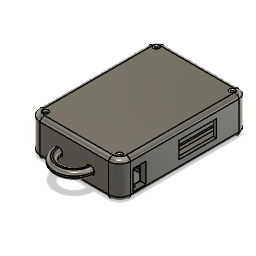
F3KStopWatch (Autodesk Fusion 360 design; units mm, degrees)
Autodesk Fusion 360 part; units mm, degrees
sketch "Sketch1" plane through (0, 0, 0) normal (0, 1, 0) x (1, 0, 0)
  line L0 (-7, 0) -> (-50, 0)
  line L1 (-57, 7) -> (-57, 75)
  line L2 (-52, 80) -> (-5, 80)
  line L3 (0, 75) -> (0, 7)
  line L4 (-57, 80) -> (0, 0) construction
  line L5 (0, 80) -> (-57, 0) construction
  line L6 (-50, 78) -> (-7, 78)
  line L7 (-2, 73) -> (-2, 9)
  line L8 (-9, 2) -> (-48, 2)
  line L9 (-55, 9) -> (-55, 73)
  line L10 (-55, 78) -> (-2, 2) construction
  line L11 (-2, 78) -> (-55, 2) construction
  line L12 (-28.5, 40) -> (-28.5, 88.1661) construction
  line L13 (-43.5, 66.1119) -> (-13.5, 66.1119)
  line L14 (-13.5, 66.1119) -> (-13.5, 26.1119)
  line L15 (-13.5, 26.1119) -> (-43.5, 26.1119)
  line L16 (-43.5, 26.1119) -> (-43.5, 66.1119)
  line L17 (-43.5, 66.1119) -> (-13.5, 26.1119) construction
  line L18 (-13.5, 66.1119) -> (-43.5, 26.1119) construction
  arc A0 (-55, 9) -> (-48, 2) centre (-48, 9) ccw
  arc A1 (-9, 2) -> (-2, 9) centre (-9, 9) ccw
  arc A2 (-2, 73) -> (-7, 78) centre (-7, 73) ccw
  arc A3 (-50, 78) -> (-55, 73) centre (-50, 73) ccw
  arc A4 (-57, 7) -> (-50, 0) centre (-50, 7) ccw
  arc A5 (-7, 0) -> (0, 7) centre (-7, 7) ccw
  arc A6 (0, 75) -> (-5, 80) centre (-5, 75) ccw
  arc A7 (-52, 80) -> (-57, 75) centre (-52, 75) ccw
  point P0 (-28.5, 40)
  point P1 (-28.5, 46.1119)
  dimension "d1" = 57
  dimension "d2" = 80
  dimension "d3" = 53
  dimension "d4" = 76
  dimension "d5" = 30
  dimension "d6" = 40
  dimension "d11" = 7
  dimension "d12" = 7
  dimension "d13" = 5
  dimension "d14" = 5
  dimension "d15" = 7
  dimension "d16" = 7
  dimension "d17" = 5
  dimension "d18" = 5
  constraint horizontal L0
  constraint vertical L1
  constraint horizontal L2
  constraint vertical L3
  constraint coincident L4.end origin
  constraint horizontal L6
  constraint perpendicular L6 L7
  constraint parallel L6 L8
  constraint parallel L7 L9
  constraint coincident L10 P0
  constraint coincident L11 P0
  constraint midpoint L4 P0
  constraint coincident P0 L12.start
  constraint perpendicular L2 L12
  constraint horizontal L13
  constraint perpendicular L13 L14
  constraint parallel L13 L15
  constraint parallel L14 L16
  constraint coincident L17 P1
  constraint coincident L18 P1
  constraint coincident L12 P1
  constraint coincident L11.end L8
  constraint coincident L11.end L9
  constraint tangent L8 A0
  constraint tangent L9 A0
  constraint coincident L10.end L8
  constraint coincident L10.end L7
  constraint tangent L8 A1
  constraint tangent L7 A1
  constraint coincident L11.start L7
  constraint coincident L11.start L6
  constraint tangent L7 A2
  constraint tangent L6 A2
  constraint coincident L10.start L9
  constraint coincident L10.start L6
  constraint tangent L9 A3
  constraint tangent L6 A3
  constraint coincident L5.end L0
  constraint coincident L5.end L1
  constraint tangent L0 A4
  constraint tangent L1 A4
  constraint coincident L4.end L0
  constraint coincident L4.end L3
  constraint tangent L0 A5
  constraint tangent L3 A5
  constraint coincident L5.start L3
  constraint coincident L5.start L2
  constraint tangent L3 A6
  constraint tangent L2 A6
  constraint coincident L4.start L1
  constraint coincident L4.start L2
  constraint tangent L1 A7
  constraint tangent L2 A7
  measures "d1" distance of L4.end L5.end
  measures "d2" distance of L4.end L5.start
  measures "d3" distance of L10.end L11.end
  measures "d4" distance of L11.start L10.end
  measures "d5" distance of L14.end L15.end
  measures "d6" distance of L13.end L14.end
  measures "d11" radius of A0
  measures "d12" radius of A1
  measures "d13" radius of A2
  measures "d14" radius of A3 P0
  measures "d15" radius of A4
  measures "d16" radius of A5
  measures "d17" radius of A6
  measures "d18" radius of A7
  measures "d154" distance of P0
  measures "d155" distance of P0
extrude "Extrude1" add sketch "Sketch1" along normal blind 2 contours L6 L7 L8 L9 A0 A1 A2 A3 makes body 1
extrude "Extrude2" add sketch "Sketch1" along normal blind 21 contours L0 L1 L2 L3 A4 A5 A6 A7 bodies 1
sketch "Sketch3" plane through (0, 0, 0) normal (0, 0, 1) x (1, 0, 0)
  circle A0 centre (40.5808, 13.4916) radius 7.15
  dimension "d19" = 14.3
  measures "d19" diameter of A0
extrude "Extrude3" add sketch "Sketch3" along normal blind 50 separate body makes body 2
move_body "Move1" bodies 2 to x (1, 0, 0) y (0, 1, 0) z (0, 0, 1) at (-26.5696, 0, -50.0846)
move_body "Move2" bodies 2 to x (0, 0, -1) y (0, 1, 0) z (1, 0, 0) at (0, 0, 0)
move_body "Move3" bodies 2 to x (1, 0, 0) y (0, 1, 0) z (0, 0, 1) at (-3.3834, 0, 1.3731)
move_body "Move4" bodies 2 to x (1, 0, 0) y (0, 1, 0) z (0, 0, 1) at (0, -5, 0)
chamfer "Chamfer1" distance 1.5 angle 45 4 edges at (-28.5, 0, -66.1119) (-13.5, 0, -46.1119) (-28.5, 0, -26.1119) (-43.5, 0, -46.1119) on bodies 1
sketch "Sketch4" plane through (0, 0, 0) normal (0, -1, 0) x (1, 0, 0)
  arc A0 (-5, -80) -> (0, -75) centre (-5, -75) ccw
  line L0 (0, -75) -> (0, -7)
  arc A1 (0, -7) -> (-7, 0) centre (-7, -7) ccw
  line L1 (-7, 0) -> (-50, 0)
  arc A2 (-50, 0) -> (-57, -7) centre (-50, -7) ccw
  line L2 (-57, -7) -> (-57, -75)
  arc A3 (-57, -75) -> (-52, -80) centre (-52, -75) ccw
  line L3 (-52, -80) -> (-5, -80)
  line L4 (-45, -24.6119) -> (-12, -24.6119)
  line L5 (-12, -24.6119) -> (-12, -67.6119)
  line L6 (-12, -67.6119) -> (-45, -67.6119)
  line L7 (-45, -67.6119) -> (-45, -24.6119)
  line L8 (-56.9925, -74.7266) -> (-56.9747, 28.4183) construction
  line L9 (0, -61.3272) -> (0, 32.8277) construction
  line L10 (-40.3582, 0) -> (-91.9722, 0) construction
  line L11 (-40.3582, 0) -> (18.5742, 0) construction
  circle A4 centre (-28.5, 0) radius 12.5
  circle A5 centre (-28.5, 0) radius 7.5
  dimension "d24" = 25
  dimension "d25" = 15
  constraint coincident A3 L8.start
  constraint coincident L0 L9.start
  constraint parallel L0 L9
  constraint coincident L1 L10.start
  constraint parallel L1 L10
  constraint perpendicular L9 L11
  constraint midpoint L1 A4.centre
  constraint concentric A4 A5
  measures "d24" diameter of A4
  measures "d25" diameter of A5
extrude "Extrude4" add sketch "Sketch4" along normal blind -13 and the other way blind 8 contours L1 A4 A5 picked at (-39.2868, 0.621) bodies 1
fillet "Fillet1" radius 3 8 edges at (-2.0503, 0, -2.0503) (-28.5, 0, 0) (-54.9497, 0, -2.0503) (-57, 0, -41) (-55.5355, 0, -78.5355) (-28.5, 0, -80) (-1.4645, 0, -78.5355) (0, 0, -41) on bodies 1
fillet "Fillet2" radius 2 8 edges at (-28.5, 2, -78) (-53.5355, 2, -76.5355) (-55, 2, -41) (-52.9497, 2, -4.0503) (-28.5, 2, -2) (-4.0503, 2, -4.0503) (-2, 2, -41) (-3.4645, 2, -76.5355) on bodies 1
fillet "Fillet3" radius 2 4 edges at (-28.5, 8, 7.5) (-28.5, 8, 12.5) (-28.5, 13, 12.5) (-28.5, 13, 7.5) on bodies 1
sketch "Sketch5" plane through (0, 2, 0) normal (0, 1, 0) x (-1, 0, 0)
  line L0 (13.5, -26.1119) -> (43.5, -26.1119)
  line L1 (43.5, -26.1119) -> (43.5, -66.1119)
  line L2 (43.5, -66.1119) -> (13.5, -66.1119)
  line L3 (13.5, -66.1119) -> (13.5, -26.1119)
  line L4 (7, -76) -> (50, -76)
  arc A0 (50, -76) -> (53, -73) centre (50, -73) ccw
  line L5 (53, -73) -> (53, -9)
  arc A1 (53, -9) -> (48, -4) centre (48, -9) ccw
  line L6 (48, -4) -> (9, -4)
  arc A2 (9, -4) -> (4, -9) centre (9, -9) ccw
  line L7 (4, -9) -> (4, -73)
  arc A3 (4, -73) -> (7, -76) centre (7, -73) ccw
  line L8 (30.7713, -66.1119) -> (30.7713, -72.1119) construction
  line L9 (30.7713, -72.1119) -> (8.1959, -72.1119) construction
  line L10 (30.7713, -72.1119) -> (48, -72.1119) construction
  line L11 (43.5, -66.1119) -> (13.5, -26.1119) construction
  line L12 (13.5, -66.1119) -> (43.5, -26.1119) construction
  line L13 (28.5, -46.1119) -> (28.5, -82.7319)
  line L14 (28.5, -46.1119) -> (28.5, -15.5457) construction
  line L15 (28.5, -72.1119) -> (10.8, -72.1119)
  line L16 (28.5, -72.1119) -> (46.2, -72.1119)
  line L17 (28.5, -26.1119) -> (28.5, -23.4119) construction
  line L18 (28.5, -23.4119) -> (46.2, -23.4119)
  line L19 (28.5, -23.4119) -> (10.8, -23.4119)
  line L20 (46.2, -72.1119) -> (46.2, -23.4119)
  line L21 (10.8, -72.1119) -> (10.8, -23.4119)
  line L22 (28.5, -22.4119) -> (9.8, -22.4119)
  line L23 (9.8, -73.1119) -> (9.8, -22.4119)
  line L24 (28.5, -73.1119) -> (9.8, -73.1119)
  line L25 (28.5, -73.1119) -> (47.2, -73.1119)
  line L26 (47.2, -73.1119) -> (47.2, -22.4119)
  line L27 (28.5, -22.4119) -> (47.2, -22.4119)
  line L28 (46.2, -72.1119) -> (42.2, -72.1119)
  line L29 (42.2, -72.1119) -> (42.2, -73.1119)
  line L30 (10.8, -72.1119) -> (15.8, -72.1119)
  line L31 (15.8, -72.1119) -> (15.8, -73.1119)
  line L32 (46.2, -23.4119) -> (41.2, -23.4119)
  line L33 (41.2, -23.4119) -> (41.2, -22.4119)
  line L34 (10.8, -23.4119) -> (15.8, -23.4119)
  line L35 (15.8, -23.4119) -> (15.8, -22.4119)
  dimension "d36" = 6
  dimension "d37" = 17.7
  dimension "d38" = 17.7
  dimension "d39" = 2.7
  dimension "d40" = 17.7
  dimension "d41" = 17.7
  dimension "d42" = 1
  dimension "d45" = 4
  dimension "d46" = 5
  dimension "d47" = 5
  dimension "d48" = 5
  constraint coincident L2 L8.start
  constraint perpendicular L2 L8
  constraint perpendicular L8 L9
  constraint perpendicular L8 L10
  constraint coincident L1.end L2.start
  constraint coincident L0.start L3.end
  constraint coincident L2.end L3.start
  constraint coincident L0.end L1.start
  constraint midpoint L11 L13.start
  constraint perpendicular L4 L13
  constraint perpendicular L0 L14
  constraint coincident L13 L15.start
  constraint coincident L9 L15.start
  constraint perpendicular L13 L15
  constraint perpendicular L8 L16
  constraint midpoint L0 L17.start
  constraint perpendicular L0 L17
  constraint perpendicular L1 L18
  constraint perpendicular L14 L19
  constraint perpendicular L20 L28
  constraint coincident L25 L29.end
  constraint perpendicular L25 L29
  constraint perpendicular L21 L30
  constraint coincident L24 L31.end
  constraint perpendicular L24 L31
  constraint perpendicular L20 L32
  constraint coincident L27 L33.end
  constraint perpendicular L27 L33
  constraint perpendicular L21 L34
  constraint coincident L22 L35.end
  constraint perpendicular L22 L35
  measures "d36" distance of L8.start L8.end
  measures "d37" distance of L15.start L15.end
  measures "d38" distance of L15.start L16.end
  measures "d39" distance of L17.start L17.end
  measures "d40" distance of L17.end L18.end
  measures "d41" distance of L17.end L19.end
  measures "d45" distance of L16.end L28.end
  measures "d46" distance of L15.end L30.end
  measures "d47" distance of L18.end L32.end
  measures "d48" distance of L19.end L34.end
extrude "Extrude5" add sketch "Sketch5" along normal blind 2 contours L13 L16 L25 L29 | L13 L15 L24 L31 | L15 L19 L21 L22 L23 L24 L30 L31 L34 L35 | L16 L18 L20 L25 L26 L27 L28 L29 L32 L33 | L18 L19 L22 L27 L33 L35 bodies 1
extrude "Extrude6" cut sketch "Sketch5" along normal blind 2 contours L13 L16 L25 L29 | L13 L15 L24 L31 | L18 L19 L22 L27 L33 L35 bodies 1
move_body "Move5" bodies 2 to x (1, 0, 0) y (0, 1, 0) z (0, 0, 1) at (0, 0.8294, 0.1037)
move_body "Move6" bodies 2 to x (1, 0, 0) y (0, 1, 0) z (0, 0, 1) at (0, 0, 0.5)
sketch "Sketch8" plane through (0, 0, 0) normal (0, 1, 0) x (1, 0, 0)
  line L0 (28.9998, 41.3515) -> (63.9998, 41.3515)
  line L1 (63.9998, 41.3515) -> (63.9998, -6.6485)
  line L2 (63.9998, -6.6485) -> (28.9998, -6.6485)
  line L3 (28.9998, -6.6485) -> (28.9998, 41.3515)
  line L4 (28.9998, 41.3515) -> (63.9998, -6.6485) construction
  line L5 (63.9998, 41.3515) -> (28.9998, -6.6485) construction
  line L6 (63.9998, -10.1485) -> (28.9998, -10.1485)
  line L7 (28.9998, -10.1485) -> (28.9998, 44.8515)
  line L8 (28.9998, 44.8515) -> (63.9998, 44.8515)
  line L9 (63.9998, 44.8515) -> (63.9998, -10.1485)
  line L10 (63.9998, -10.1485) -> (28.9998, 44.8515) construction
  line L11 (28.9998, -10.1485) -> (63.9998, 44.8515) construction
  line L12 (56.9998, -8.6485) -> (35.9998, -8.6485)
  line L13 (35.9998, -8.6485) -> (35.9998, 43.3515)
  line L14 (35.9998, 43.3515) -> (56.9998, 43.3515)
  line L15 (56.9998, 43.3515) -> (56.9998, -8.6485)
  line L16 (56.9998, -8.6485) -> (35.9998, 43.3515) construction
  line L17 (35.9998, -8.6485) -> (56.9998, 43.3515) construction
  point P0 (46.4998, 17.3515)
  point P1 (46.4998, 17.3515)
  dimension "d63" = 35
  dimension "d64" = 48
  dimension "d65" = 35
  dimension "d66" = 55
  dimension "d67" = 21
  dimension "d68" = 52
  constraint horizontal L0
  constraint vertical L1
  constraint horizontal L2
  constraint vertical L3
  constraint horizontal L6
  constraint perpendicular L6 L7
  constraint parallel L6 L8
  constraint parallel L7 L9
  constraint coincident L10 P1
  constraint coincident L11 P1
  constraint midpoint L5 P1
  constraint horizontal L12
  constraint perpendicular L12 L13
  constraint parallel L12 L14
  constraint parallel L13 L15
  constraint coincident L16 P1
  constraint coincident L17 P1
  constraint coincident P1 P0
  measures "d63" distance of L0.start L0.end
  measures "d64" distance of L0.start L2.end
  measures "d65" distance of L7.end L8.end
  measures "d66" distance of L6.end L7.end
  measures "d67" distance of L13.end L14.end
  measures "d68" distance of L12.end L13.end
extrude "Extrude8" add sketch "Sketch8" along normal blind 16.5 and the other way blind -3.1 separate body contours L0 L13 L14 L15 | L0 L2 L13 L15 | L2 L12 L13 L15 makes body 3
extrude "Extrude9" add sketch "Sketch8" along normal blind 3.1 separate body contours L0 L2 L3 L7 L13 | L0 L2 L13 L15 | L0 L1 L2 L9 L15 makes body 4
extrude "Extrude10" add sketch "Sketch8" along normal blind 4.9 and the other way blind -3.1 separate body makes body 5
combine "Combine1" operation add target body 3 tool bodies 4 5 keep tools
combine "Combine2" operation add target body 4 tool bodies 3 5 keep tools
combine "Combine3" operation add target body 3 tool bodies 4 5 keep tools
combine "Combine4" operation add target body 3 tool bodies 5 keep tools
combine "Combine5" operation add target body 3 tool bodies 4 keep tools
delete_body "RemoveBody1" bodies 4
delete_body "RemoveBody2" bodies 5
move_body "Move7" bodies 3 to x (1, 0, 0) y (0, 1, 0) z (0, 0, 1) at (-75.2922, 0, -30.8262)
move_body "Move8" bodies 3 to x (1, 0, 0) y (0, 1, 0) z (0, 0, 1) at (0, 2, 0)
move_body "Move9" bodies 3 to x (1, 0, 0) y (0, 1, 0) z (0, 0, 1) at (0, 0, 0.4)
move_body "Move10" bodies 3 to x (1, 0, 0) y (0, 1, 0) z (0, 0, 1) at (0.3, 0, 0)
move_body "Move11" bodies 2 to x (0, 0, 1) y (0, 1, 0) z (-1, 0, 0) at (0, 0, 0)
move_body "Move12" bodies 2 to x (1, 0, 0) y (0, 1, 0) z (0, 0, 1) at (-58.8123, 0, -12.8386)
move_body "Move13" bodies 2 to x (1, 0, 0) y (0, 1, 0) z (0, 0, 1) at (-1.1, 4.5, 0)
sketch "Sketch9" plane through (0, 0, 0) normal (1, 0, 0) x (0, 0, -1)
  line L0 (7, 3) -> (75, 3)
  line L1 (75, 3) -> (75, 21)
  line L2 (75, 21) -> (7, 21)
  line L3 (7, 21) -> (7, 3)
  line L4 (75, 12) -> (49, 12) construction
  line L5 (60.75, 6.75) -> (37.25, 6.75)
  line L6 (37.25, 6.75) -> (37.25, 17.25)
  line L7 (37.25, 17.25) -> (60.75, 17.25)
  line L8 (60.75, 17.25) -> (60.75, 6.75)
  line L9 (60.75, 6.75) -> (37.25, 17.25) construction
  line L10 (37.25, 6.75) -> (60.75, 17.25) construction
  point P0 (49, 12)
  dimension "d80" = 26
  dimension "d81" = 23.5
  dimension "d82" = 10.5
  constraint midpoint L1 L4.start
  constraint perpendicular L1 L4
  constraint horizontal L5
  constraint perpendicular L5 L6
  constraint parallel L5 L7
  constraint parallel L6 L8
  constraint coincident L9 P0
  constraint coincident L10 P0
  constraint coincident P0 L4.end
  measures "d80" distance of L4.start P0
  measures "d81" distance of L6.end L7.end
  measures "d82" distance of L5.end L6.end
extrude "Extrude11" cut sketch "Sketch9" against normal blind 3 contours L5 L6 L7 L8 bodies 1
sketch "Sketch10" plane through (0, 2, 0) normal (0, 1, 0) x (-1, 0, 0)
  line L0 (41.2, -22.4119) -> (47.2, -22.4119)
  line L1 (47.2, -22.4119) -> (47.2, -73.1119)
  line L2 (47.2, -73.1119) -> (42.2, -73.1119)
  line L3 (42.2, -73.1119) -> (42.2, -72.1119)
  line L4 (42.2, -72.1119) -> (46.2, -72.1119)
  line L5 (46.2, -72.1119) -> (46.2, -23.4119)
  line L6 (46.2, -23.4119) -> (41.2, -23.4119)
  line L7 (41.2, -23.4119) -> (41.2, -22.4119)
  line L8 (13.5, -26.1119) -> (43.5, -26.1119)
  line L9 (43.5, -26.1119) -> (43.5, -66.1119)
  line L10 (43.5, -66.1119) -> (13.5, -66.1119)
  line L11 (13.5, -66.1119) -> (13.5, -26.1119)
  line L12 (7, -76) -> (50, -76)
  arc A0 (50, -76) -> (53, -73) centre (50, -73) ccw
  line L13 (53, -73) -> (53, -9)
  arc A1 (53, -9) -> (48, -4) centre (48, -9) ccw
  line L14 (48, -4) -> (9, -4)
  arc A2 (9, -4) -> (4, -9) centre (9, -9) ccw
  line L15 (4, -9) -> (4, -73)
  arc A3 (4, -73) -> (7, -76) centre (7, -73) ccw
  line L16 (15.8, -22.4119) -> (15.8, -23.4119)
  line L17 (15.8, -23.4119) -> (10.8, -23.4119)
  line L18 (10.8, -23.4119) -> (10.8, -72.1119)
  line L19 (10.8, -72.1119) -> (15.8, -72.1119)
  line L20 (15.8, -72.1119) -> (15.8, -73.1119)
  line L21 (15.8, -73.1119) -> (9.8, -73.1119)
  line L22 (9.8, -73.1119) -> (9.8, -22.4119)
  line L23 (9.8, -22.4119) -> (15.8, -22.4119)
  line L24 (42.4256, -4) -> (42.4256, -16.2447) construction
  line L25 (50.4256, -6.1223) -> (34.4256, -6.1223)
  line L26 (34.4256, -6.1223) -> (34.4256, -14.1223)
  line L27 (34.4256, -14.1223) -> (50.4256, -14.1223)
  line L28 (50.4256, -14.1223) -> (50.4256, -6.1223)
  line L29 (50.4256, -6.1223) -> (34.4256, -14.1223) construction
  line L30 (34.4256, -6.1223) -> (50.4256, -14.1223) construction
  point P0 (42.4256, -10.1223)
  dimension "d85" = 16
  dimension "d86" = 8
  constraint coincident L14 L24.start
  constraint perpendicular L14 L24
  constraint horizontal L25
  constraint perpendicular L25 L26
  constraint parallel L25 L27
  constraint parallel L26 L28
  constraint coincident L29 P0
  constraint coincident L30 P0
  constraint midpoint L24 P0
  measures "d85" distance of L26.end L27.end
  measures "d86" distance of L25.end L26.end
extrude "Extrude12" cut sketch "Sketch10" against normal blind 9 contours L25 L26 L27 L28 bodies 1
sketch "Sketch15" plane through (0, 2, 0) normal (0, 1, 0) x (-1, 0, 0)
  line L0 (34.4256, -6.1223) -> (50.4256, -6.1223)
  line L1 (50.4256, -6.1223) -> (50.4256, -14.1223)
  line L2 (50.4256, -14.1223) -> (34.4256, -14.1223)
  line L3 (34.4256, -14.1223) -> (34.4256, -6.1223)
  line L4 (41.2, -22.4119) -> (47.2, -22.4119)
  line L5 (47.2, -22.4119) -> (47.2, -73.1119)
  line L6 (47.2, -73.1119) -> (42.2, -73.1119)
  line L7 (42.2, -73.1119) -> (42.2, -72.1119)
  line L8 (42.2, -72.1119) -> (46.2, -72.1119)
  line L9 (46.2, -72.1119) -> (46.2, -23.4119)
  line L10 (46.2, -23.4119) -> (41.2, -23.4119)
  line L11 (41.2, -23.4119) -> (41.2, -22.4119)
  line L12 (13.5, -26.1119) -> (43.5, -26.1119)
  line L13 (43.5, -26.1119) -> (43.5, -66.1119)
  line L14 (43.5, -66.1119) -> (13.5, -66.1119)
  line L15 (13.5, -66.1119) -> (13.5, -26.1119)
  line L16 (7, -76) -> (50, -76)
  arc A0 (50, -76) -> (53, -73) centre (50, -73) ccw
  line L17 (53, -73) -> (53, -9)
  arc A1 (53, -9) -> (48, -4) centre (48, -9) ccw
  line L18 (48, -4) -> (9, -4)
  arc A2 (9, -4) -> (4, -9) centre (9, -9) ccw
  line L19 (4, -9) -> (4, -73)
  arc A3 (4, -73) -> (7, -76) centre (7, -73) ccw
  line L20 (15.8, -22.4119) -> (15.8, -23.4119)
  line L21 (15.8, -23.4119) -> (10.8, -23.4119)
  line L22 (10.8, -23.4119) -> (10.8, -72.1119)
  line L23 (10.8, -72.1119) -> (15.8, -72.1119)
  line L24 (15.8, -72.1119) -> (15.8, -73.1119)
  line L25 (15.8, -73.1119) -> (9.8, -73.1119)
  line L26 (9.8, -73.1119) -> (9.8, -22.4119)
  line L27 (9.8, -22.4119) -> (15.8, -22.4119)
  line L28 (4, -9) -> (31.5949, -9) construction
  line L29 (4, -9) -> (-8.1404, -9) construction
  line L30 (4, -9) -> (25, -9)
  line L31 (25, -9) -> (25, -1.0306)
  line L32 (4, -9) -> (2.2, -9)
  line L33 (25, -1.0306) -> (-6.9566, -1.0306) construction
  line L34 (2.2, -9) -> (2.2, -7.0306)
  line L35 (2.2, -1.0306) -> (25, -1.0306)
  line L36 (25, -1.0306) -> (8.2, -1.0306)
  arc A4 (8.2, -1.0306) -> (2.2, -7.0306) centre (8.2, -7.0306) ccw
  dimension "d107" = 21
  dimension "d113" = 1.8
  dimension "d114" = 6
  constraint coincident A2.end L19.start
  constraint perpendicular L19 L28
  constraint perpendicular L19 L29
  constraint perpendicular L19 L30
  constraint perpendicular L18 L31
  constraint perpendicular L19 L32
  constraint perpendicular L31 L33
  constraint coincident L33 L35.start
  constraint perpendicular L33 L34
  constraint coincident L35.start L34
  constraint coincident L35.start L36
  constraint tangent L34 A4
  constraint tangent L36 A4
  measures "d107" distance of A2.end L30.end
  measures "d113" distance of A2.end L32.end
  measures "d114" radius of A4
extrude "Extrude18" add sketch "Sketch15" along normal blind 18 separate body contours L18 A2 L31 L32 L34 L35 L36 A4 | L18 A2 L30 L31 makes body 6
move_body "Move14" bodies 6 to x (1, 0, 0) y (0, 1, 0) z (0, 0, 1) at (2, 0, 0)
fillet "Fillet7" [no effect]
combine "Combine7" operation add target body 1 tool bodies 6 keep tools
delete_body "RemoveBody3" bodies 6
fillet "Fillet8" radius 1 5 edges at (-23, 11, -9) (-23, 12, -2) (-23, 2.5858, -2.5858) (-23, 2, -6.5) (-23, 20, -5.5) on bodies 1
fillet "Fillet9" radius 1 2 edges at (-12, 20, -9) (-22.7071, 19.7071, -8.7071) on bodies 1
sketch "Sketch16" plane through (-2, 0, 0) normal (-1, 0, 0) x (0, 0, 1)
  line L0 (-37.25, 17.25) -> (-37.25, 6.75)
  line L1 (-37.25, 6.75) -> (-60.75, 6.75)
  line L2 (-60.75, 6.75) -> (-60.75, 17.25)
  line L3 (-60.75, 17.25) -> (-37.25, 17.25)
  line L4 (-73, 4) -> (-9, 4)
  line L5 (-9, 4) -> (-9, 19)
  line L6 (-9, 19) -> (-9, 21)
  line L7 (-9, 21) -> (-73, 21)
  line L8 (-73, 21) -> (-73, 4)
  line L9 (-9, -0.9635) -> (-9, 21) construction
  line L10 (-9, 10.0182) -> (-22.3565, 10.0182) construction
  line L11 (-9, 10.0182) -> (-10.5, 10.0182) construction
  line L12 (-10.5, 10.0182) -> (-14.5, 10.0182) construction
  line L13 (-14.5, 10.0182) -> (-12.5, 10.0182) construction
  line L14 (-14.75, 14.5182) -> (-10.25, 14.5182)
  line L15 (-10.25, 14.5182) -> (-10.25, 5.5182)
  line L16 (-10.25, 5.5182) -> (-14.75, 5.5182)
  line L17 (-14.75, 5.5182) -> (-14.75, 14.5182)
  line L18 (-14.75, 14.5182) -> (-10.25, 5.5182) construction
  line L19 (-10.25, 14.5182) -> (-14.75, 5.5182) construction
  point P0 (-12.5, 10.0182)
  dimension "d119" = 13.3565
  dimension "d120" = 1.5
  dimension "d121" = 4
  dimension "d122" = 4.5
  dimension "d123" = 9
  constraint coincident L6.end L7.start
  constraint perpendicular L7 L9
  constraint midpoint L9 L10.start
  constraint perpendicular L9 L10
  constraint perpendicular L5 L11
  constraint perpendicular L9 L12
  constraint midpoint L12 P0
  constraint horizontal L14
  constraint perpendicular L14 L15
  constraint parallel L14 L16
  constraint parallel L15 L17
  constraint coincident L18 P0
  constraint coincident L19 P0
  constraint coincident P0 L13.end
  measures "d119" distance of L10.start L10.end
  measures "d120" distance of L10.start L11.end
  measures "d121" distance of L11.end L12.end
  measures "d122" distance of L15.end L16.end
  measures "d123" distance of L14.end L15.end
extrude "Extrude19" cut sketch "Sketch16" against normal blind 4 contours L14 L15 L16 L17 bodies 1
chamfer "Chamfer2" distance 1.8 angle 45 4 edges at (0, 14.5182, -12.5) (0, 10.0182, -14.75) (0, 5.5182, -12.5) (0, 10.0182, -10.25) on bodies 1
sketch "Sketch17" plane through (0, 0, -2) normal (0, 0, -1) x (-1, 0, 0)
  line L0 (24, 19) -> (24, 4)
  line L1 (24, 4) -> (48, 4)
  line L2 (48, 4) -> (48, 21)
  line L3 (48, 21) -> (9, 21)
  line L4 (9, 21) -> (9, 20)
  line L5 (9, 20) -> (22.2679, 20)
  spline S0 degree 3 poles (22.2679, 20) (22.5228, 20) (22.8153, 19.9104) (23.3848, 19.6039) (23.7229, 19.2771) (24, 19) knots 0.505532 0.505532 0.505532 0.505532 0.581995 0.581995 0.699558 0.699558 0.699558 0.699558
  line L6 (55.8373, 1.7757) -> (46.5836, 1.7757)
  line L7 (46.5836, 1.7757) -> (46.5836, 12.5)
  line L8 (46.5836, 12.5) -> (55.8373, 12.5)
  line L9 (55.8373, 12.5) -> (55.8373, 1.7757)
  dimension "d127" = 9.2536
  constraint horizontal L6
  constraint vertical L7
  constraint horizontal L8
  constraint vertical L9
  measures "d127" distance of L6.start L6.end
extrude "Extrude20" add sketch "Sketch17" along normal blind 65.5 and the other way blind -13 separate body contours L1 L2 L7 L8 | L1 L2 L6 L7 L8 L9 makes body 7
combine "Combine8" operation cut target body 7 tool bodies 2 keep tools
combine "Combine9" operation add target body 1 tool bodies 7 keep tools
delete_body "RemoveBody4" bodies 7
sketch "Sketch18" plane through (0, 2, 0) normal (0, 1, 0) x (-1, 0, 0)
  line L0 (1.0146, -8.9828) -> (25.0146, -8.9828)
  line L1 (25.0146, -8.9828) -> (25.0146, -10.7828)
  line L2 (25.0146, -10.7828) -> (1.0146, -10.7828)
  line L3 (1.0146, -10.7828) -> (1.0146, -8.9828)
  dimension "d132" = 24
  dimension "d133" = 1.8
  constraint horizontal L0
  constraint vertical L1
  constraint horizontal L2
  constraint vertical L3
  measures "d132" distance of L0.start L0.end
  measures "d133" distance of L0.start L2.end
extrude "Extrude21" cut sketch "Sketch18" along normal blind 23 and the other way blind 0 bodies 1
sketch "Sketch19" plane through (0, 0, -80) normal (0, 0, -1) x (-1, 0, 0)
  line L0 (5, 3) -> (52, 3)
  line L1 (52, 3) -> (52, 21)
  line L2 (52, 21) -> (5, 21) construction
  line L3 (5, 21) -> (5, 3)
  line L4 (5, 12) -> (52, 12) construction
  line L5 (5, 12) -> (13, 12)
  line L6 (52, 12) -> (44, 12)
  circle A0 centre (13, 12) radius 6.25
  circle A1 centre (13, 12) radius 8.75 construction
  circle A2 centre (44, 12) radius 8.75 construction
  circle A3 centre (44, 12) radius 6.25
  dimension "d138" = 8
  dimension "d139" = 8
  dimension "d140" = 12.5
  dimension "d141" = 17.5
  dimension "d142" = 17.5
  dimension "d143" = 12.5
  constraint midpoint L3 L4.start
  constraint midpoint L1 L4.end
  constraint perpendicular L3 L5
  constraint perpendicular L1 L6
  constraint coincident L5.end A0.centre
  constraint concentric A0 A1
  constraint coincident L6.end A2.centre
  constraint concentric A2 A3
  measures "d138" distance of L4.start L5.end
  measures "d139" distance of L4.end L6.end
  measures "d140" diameter of A0
  measures "d141" diameter of A1
  measures "d142" diameter of A2
  measures "d143" diameter of A3
extrude "Extrude22" cut sketch "Sketch19" against normal blind 3 bodies 1
sketch "Sketch20" plane through (0, 21, 0) normal (0, 1, 0) x (-1, 0, 0)
  arc A0 (0, -75) -> (5, -80) centre (5, -75) ccw
  line L0 (5, -80) -> (52, -80)
  arc A1 (52, -80) -> (57, -75) centre (52, -75) ccw
  line L1 (57, -75) -> (57, -7)
  arc A2 (57, -7) -> (50, 0) centre (50, -7) ccw
  line L2 (50, 0) -> (7, 0)
  arc A3 (7, 0) -> (0, -7) centre (7, -7) ccw
  line L3 (0, -7) -> (0, -75)
  line L4 (2, -10.7828) -> (1.0146, -10.7828)
  line L5 (1.0146, -10.7828) -> (1.0146, -8.9828)
  line L6 (1.0146, -8.9828) -> (2, -8.9828)
  arc A4 (9, -2) -> (2, -8.9828) centre (9, -9) ccw
  line L7 (9, -2) -> (48, -2)
  arc A5 (55, -9) -> (48, -2) centre (48, -9) ccw
  line L8 (55, -9) -> (55, -73)
  arc A6 (50, -78) -> (55, -73) centre (50, -73) ccw
  line L9 (50, -78) -> (7, -78)
  arc A7 (2, -73) -> (7, -78) centre (7, -73) ccw
  line L10 (2, -73) -> (2, -10.7828)
extrude "Extrude23" add sketch "Sketch20" along normal blind 2 and the other way blind 1 separate body contours A0 L0 A1 L1 A2 L2 A3 L3 | L4 L5 L6 A4 L7 A5 L8 A6 L9 A7 L10 makes body 8
combine "Combine10" operation cut target body 8 tool bodies 1 2 keep tools
fillet "Fillet11" radius 3 8 edges at (-57, 23, -41) (-54.9497, 23, -2.0503) (-28.5, 23, 0) (-2.0503, 23, -2.0503) (0, 23, -41) (-1.4645, 23, -78.5355) (-28.5, 23, -80) (-55.5355, 23, -78.5355) on bodies 8
sketch "Sketch21" plane through (0, 21, 0) normal (0, 1, 0) x (-1, 0, 0)
  arc A0 (0, -75) -> (5, -80) centre (5, -75) ccw
  line L0 (5, -80) -> (52, -80)
  arc A1 (52, -80) -> (57, -75) centre (52, -75) ccw
  line L1 (57, -75) -> (57, -7)
  arc A2 (57, -7) -> (50, 0) centre (50, -7) ccw
  line L2 (50, 0) -> (7, 0)
  arc A3 (7, 0) -> (0, -7) centre (7, -7) ccw
  line L3 (0, -7) -> (0, -75)
  line L4 (2, -10.7828) -> (1.0146, -10.7828)
  line L5 (1.0146, -10.7828) -> (1.0146, -8.9828)
  line L6 (1.0146, -8.9828) -> (2, -8.9828)
  arc A4 (9, -2) -> (2, -8.9828) centre (9, -9) ccw
  line L7 (9, -2) -> (48, -2)
  arc A5 (55, -9) -> (48, -2) centre (48, -9) ccw
  line L8 (55, -9) -> (55, -73)
  arc A6 (50, -78) -> (55, -73) centre (50, -73) ccw
  line L9 (50, -78) -> (7, -78)
  arc A7 (2, -73) -> (7, -78) centre (7, -73) ccw
  line L10 (2, -73) -> (2, -10.7828)
  line L11 (0.9141, -73) -> (4, -73)
  line L12 (7, -76) -> (7, -78.5355)
  line L13 (7, -78.5355) -> (5.9141, -78.5355)
  line L14 (0.9141, -73.5355) -> (0.9141, -73)
  line L15 (50, -78.5355) -> (51, -78.5355)
  line L16 (56, -73.5355) -> (56, -72.5355)
  line L17 (56, -72.5355) -> (53, -72.5355)
  line L18 (50, -75.5355) -> (50, -78.5355)
  line L19 (55.8559, -7.968) -> (54.2906, -7.968)
  line L20 (48.7906, -2.468) -> (48.7906, -0.9027)
  line L21 (48.7906, -0.9027) -> (48.3559, -0.9027)
  line L22 (55.8559, -8.4027) -> (55.8559, -7.968)
  arc A8 (0.9141, -73.5355) -> (5.9141, -78.5355) centre (5.9141, -73.5355) ccw
  arc A9 (51, -78.5355) -> (56, -73.5355) centre (51, -73.5355) ccw
  arc A10 (55.8559, -8.4027) -> (48.3559, -0.9027) centre (48.3559, -8.4027) ccw
  arc A11 (48.7906, -2.468) -> (54.2906, -7.968) centre (54.2906, -2.468) ccw
  arc A12 (53, -72.5355) -> (50, -75.5355) centre (53, -75.5355) ccw
  arc A13 (7, -76) -> (4, -73) centre (4, -76) ccw
  point P0 (56, -78.5355)
  point P1 (50, -72.5355)
  point P2 (48.7906, -7.968)
  dimension "d154" = 6
  dimension "d155" = 6
  dimension "d156" = 7.0653
  dimension "d157" = 5
  dimension "d158" = 5
  dimension "d159" = 7.5
  dimension "d160" = 5.5
  dimension "d161" = 3
  dimension "d162" = 3
  constraint horizontal L11
  constraint vertical L12
  constraint horizontal L13
  constraint vertical L14
  constraint horizontal L15
  constraint vertical L16
  constraint horizontal L17
  constraint vertical L18
  constraint horizontal L19
  constraint vertical L20
  constraint horizontal L21
  constraint vertical L22
  constraint tangent L13 A8
  constraint tangent L14 A8
  constraint coincident P0 L15
  constraint coincident P0 L16
  constraint tangent L15 A9
  constraint tangent L16 A9
  constraint tangent L21 A10
  constraint tangent L22 A10
  constraint coincident P2 L20
  constraint coincident P2 L19
  constraint tangent L20 A11
  constraint tangent L19 A11
  constraint coincident P1 L17
  constraint coincident P1 L18
  constraint tangent L17 A12
  constraint tangent L18 A12
  constraint tangent L11 A13
  constraint tangent L12 A13
  measures "d154" distance of L15.start P0
  measures "d155" distance of L15.start P1
  measures "d156" distance of L19.start P2
  measures "d157" radius of A8
  measures "d158" radius of A9
  measures "d159" radius of A10
  measures "d160" radius of A11
  measures "d161" radius of A12
  measures "d162" radius of A13
extrude "Extrude24" add sketch "Sketch21" along normal blind -7 and the other way blind 1 contours A7 L11 L12 A13 bodies 1
extrude "Extrude25" add sketch "Sketch21" along normal blind -6 and the other way blind 1 contours L8 A6 L17 L18 A12 bodies 1
extrude "Extrude26" add sketch "Sketch21" along normal blind -7 and the other way blind 1 contours A5 L19 L20 A11 bodies 1
fillet "Fillet12" radius 2 9 edges at (-54.6071, 14, -7.968) (-50.4015, 14, -6.3571) (-48.7906, 14, -2.2564) (-3, 14, -73) (-6.1213, 14, -73.8787) (-7, 14, -77) (-50, 15, -76.7678) (-50.8787, 15, -73.4142) (-54, 15, -72.5355) on bodies 1
fillet "Fillet13" radius 1 4 edges at (-50.7918, 12.5, -15) (-46.5836, 7.25, -15) (-50.7918, 12.5, -67.5) (-46.5836, 8.25, -67.5) on bodies 1
sketch "Sketch22" plane through (0, 2, 0) normal (0, 1, 0) x (-1, 0, 0)
  line L0 (4, -10.7828) -> (4, -73)
  arc A0 (4, -73) -> (7, -76) centre (7, -73) ccw
  line L1 (7, -76) -> (50, -76)
  arc A1 (50, -76) -> (53, -73) centre (50, -73) ccw
  line L2 (53, -73) -> (53, -67.5)
  line L3 (53, -67.5) -> (47.5836, -67.5)
  arc A2 (47.2, -67.4235) -> (47.5836, -67.5) centre (47.5836, -66.5) ccw
  line L4 (47.2, -67.4235) -> (47.2, -73.1119)
  line L5 (47.2, -73.1119) -> (42.2, -73.1119)
  line L6 (42.2, -73.1119) -> (42.2, -72.1119)
  line L7 (42.2, -72.1119) -> (46.2, -72.1119)
  line L8 (46.2, -72.1119) -> (46.2, -23.4119)
  line L9 (46.2, -23.4119) -> (41.2, -23.4119)
  line L10 (41.2, -23.4119) -> (41.2, -22.4119)
  line L11 (41.2, -22.4119) -> (46.5836, -22.4119)
  line L12 (46.5836, -22.4119) -> (46.5836, -16)
  arc A3 (47.5836, -15) -> (46.5836, -16) centre (47.5836, -16) ccw
  line L13 (47.5836, -15) -> (53, -15)
  line L14 (53, -15) -> (53, -9)
  arc A4 (53, -9) -> (48, -4) centre (48, -9) ccw
  line L15 (48, -4) -> (24, -4)
  line L16 (24, -4) -> (24, -8)
  spline S0 degree 3 poles (24, -8) (23.7229, -8.2771) (23.3848, -8.6039) (22.8771, -8.8772) (22.6793, -8.9523) (22.4851, -8.9828) knots 0 0 0 0 0.117563 0.117563 0.172976 0.172976 0.172976 0.172976
  line L17 (22.4851, -8.9828) -> (1.0146, -8.9828)
  line L18 (1.0146, -8.9828) -> (1.0146, -10.7828)
  line L19 (1.0146, -10.7828) -> (4, -10.7828)
  line L20 (15.8, -22.4119) -> (15.8, -23.4119)
  line L21 (15.8, -23.4119) -> (10.8, -23.4119)
  line L22 (10.8, -23.4119) -> (10.8, -72.1119)
  line L23 (10.8, -72.1119) -> (15.8, -72.1119)
  line L24 (15.8, -72.1119) -> (15.8, -73.1119)
  line L25 (15.8, -73.1119) -> (9.8, -73.1119)
  line L26 (9.8, -73.1119) -> (9.8, -22.4119)
  line L27 (9.8, -22.4119) -> (15.8, -22.4119)
  line L28 (13.5, -26.1119) -> (43.5, -26.1119)
  line L29 (43.5, -26.1119) -> (43.5, -66.1119)
  line L30 (43.5, -66.1119) -> (13.5, -66.1119)
  line L31 (13.5, -66.1119) -> (13.5, -26.1119)
  line L32 (34.4256, -6.1223) -> (50.4256, -6.1223)
  line L33 (50.4256, -6.1223) -> (50.4256, -14.1223)
  line L34 (50.4256, -14.1223) -> (34.4256, -14.1223)
  line L35 (34.4256, -14.1223) -> (34.4256, -6.1223)
  line L36 (4, -10.7828) -> (23.8799, -10.7828) construction
  line L37 (1.0146, -10.7828) -> (14.0146, -10.7828) construction
  line L38 (14.0146, -10.7828) -> (19.0146, -10.7828)
  line L39 (19.0146, -10.7828) -> (19.0146, -11.7828)
  line L40 (19.0146, -11.7828) -> (14.0146, -11.7828)
  line L41 (14.0146, -11.7828) -> (14.0146, -10.7828)
  dimension "d179" = 13
  dimension "d180" = 5
  dimension "d181" = 1
  constraint coincident L0.start L19.end
  constraint perpendicular L0 L36
  constraint coincident L18.end L19.start
  constraint perpendicular L18 L37
  constraint horizontal L38
  constraint vertical L39
  constraint horizontal L40
  constraint vertical L41
  measures "d179" distance of L18.end L37.end
  measures "d180" distance of L37.end L38.end
  measures "d181" distance of L37.end L40.end
extrude "Extrude27" add sketch "Sketch22" along normal blind 1 contours L38 L39 L40 L41 bodies 1
hole "Hole1" at (-51.5948, 23, -5.2565) direction (0, -1, 0) diameter 2 depth 3 tip angle 118 countersink diameter 3.5 countersink angle 90 bodies 8
hole "Hole2" at (-5.3341, 23, -5.2152) direction (0, -1, 0) diameter 2 depth 3 tip angle 118 countersink diameter 3.5 countersink angle 90 bodies 8
hole "Hole3" at (-4.6435, 23, -75.3425) direction (0, -1, 0) diameter 2 depth 3 tip angle 118 countersink diameter 3.5 countersink angle 90 bodies 8
hole "Hole4" at (-52.3083, 23, -75.2725) direction (0, -1, 0) diameter 2 depth 3 tip angle 118 countersink diameter 3.5 countersink angle 90 bodies 8
hole "Hole6" at (-4.7682, 20, -75.3197) direction (0, -1, 0) diameter 1 depth 6 tip angle 118 bodies 1
hole "Hole7" at (-52.2905, 20, -75.2757) direction (0, -1, 0) diameter 1 depth 6 tip angle 118 bodies 1
hole "Hole8" at (-51.59, 20, -5.265) direction (0, -1, 0) diameter 1 depth 6 tip angle 118 bodies 1
hole "Hole9" at (-5.325, 20, -5.2026) direction (0, -1, 0) diameter 1 depth 6 tip angle 118 bodies 1
move_face "OffsetFaces1" offset -0.5 11 faces at (-2.1409, 20.3333, -74.1788) (-35.6667, 20.6667, -78) (-2, 20.6667, -52.2609) (-1.6715, 20.3333, -10.7828) (-3.5038, 20.3333, -4.6651) (-1.0146, 20.3333, -10.1828) (-50.4753, 20.3333, -77.9774) (-55, 20.6667, -30.3333) (-51.5, 20.3333, -2.9378) (-22, 20.3333, -2) (-1.3431, 20.3333, -8.9828) on bodies 8
named bodies: "Case", "Battery", "Pico", "Back"
